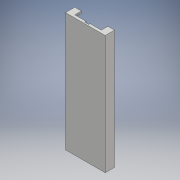
# Autodesk Inventor part: Base
Saved by Autodesk Inventor 2017 (Build 210142000, 142)
## iProperties
Created: 2017-01-18
Part Number: Base
Material: Generic
Document SubType Name: Modeling
Designer: A. Matías Quezada
Density: 1 g/cm^3
Appearance: Default
Author: A. Matías Quezada
Autodesk Inventor part; units mm, degrees
ref_plane "YZ Plane" through (0, 0, 0) normal (1, 0, 0) x (0, 1, 0)
ref_plane "XZ Plane" through (0, 0, 0) normal (0, 1, 0) x (-1, 0, 0)
ref_plane "XY Plane" through (0, 0, 0) normal (0, 0, 1) x (1, 0, 0)
sketch "Sketch1" plane through (0, 0, 0) normal (0, 1, 0) x (-1, 0, 0)
  line L0 (0, 0) -> (60, 0)
  line L1 (60, 0) -> (60, 180)
  line L2 (60, 180) -> (0, 180)
  line L3 (0, 180) -> (0, 0)
  dimension "d1" = 60
  dimension "d2" = 180
  constraints: 8 end point, 2 parallel, 1 horizontal, 1 perpendicular
  measures "d1" distance of L2.end L1.end
  measures "d2" distance of L1.end L0.end
extrude "Base" add sketch "Sketch1" along normal blind 4
sketch "Sketch3" plane through (0, 4, 0) normal (0, 1, 0) x (1, 0, 0)
  line L0 (-60, 0) -> (-60, -180) projected
  line L1 (-60, -180) -> (0, -180) projected
  line L2 (0, -180) -> (0, 0) projected
  line L3 (0, 0) -> (-60, 0) projected
  line L4 (-57, -177) -> (-57, -3)
  line L5 (-57, -3) -> (-3, -3)
  line L6 (-3, -3) -> (-3, -177)
  line L7 (-3, -177) -> (-57, -177)
  line L8 (-30, -198.6939) -> (-30, 11.8917)
  line L9 (-50, -180) -> (-10, -180)
  line L10 (-10, -180) -> (-10, -177)
  line L11 (-10, -177) -> (-50, -177)
  line L12 (-50, -177) -> (-50, -180)
  point P0 (-30, 0)
  point P1 (-30, -180)
  point P2 (-30, -177)
  dimension "d10" = 3
  dimension "d11" = 40
  constraints: 18 end point, 5 midpoint, 2 parallel, 1 horizontal, 1 perpendicular, 1 point on line, 1 vertical, 3 other
  measures "d10" distance between parallel lines of L0 L4
  measures "d11" distance between parallel lines of L10 L12
extrude "Muros" add sketch "Sketch3" along normal blind 10 contours L3 L8 L5 L4 L7 L12 L1 L0 | L3 L2 L1 L10 L7 L6 L5 L8
sketch "Sketch4" plane through (0, 4, 0) normal (0, 1, 0) x (1, 0, 0)
  line L0 (-50, -180) -> (-10, -180) projected
  line L1 (-57, -3) -> (-3, -3) projected
  line L2 (-33, -180) -> (-27, -180)
  line L3 (-27, -180) -> (-27, -3)
  line L4 (-27, -3) -> (-33, -3)
  line L5 (-33, -3) -> (-33, -180)
  line L6 (-3, -3) -> (-57, -3) projected
  point P0 (0, 0)
  point P1 (-30, -3)
  point P2 (-30, -3)
  point P3 (-30, -180)
  dimension "d14" = 6
  constraints: 8 end point, 5 midpoint, 2 parallel, 1 horizontal, 1 perpendicular
  measures "d14" distance between parallel lines of L3 L5
extrude "Rail" cut sketch "Sketch4" against normal blind 2
equation "\"d1\" = base_base_ancho"
equation "\"d2\" = base_base_largo"
equation "\"d4\" = base_base_grosor"
equation "\"d10\" = base_muros_grosor"
equation "\"d11\" = base_muros_separación"
equation "\"d12\" = base_muros_alto"
equation "\"d14\" = base_rail_ancho"
equation "\"d15\" = base_rail_profundidad"
equation "\"base_base_ancho\" = 60"
equation "\"base_base_largo\" = 180"
equation "\"base_base_grosor\" = 4"
equation "\"base_muros_grosor\" = 3"
equation "\"base_muros_separación\" = 40"
equation "\"base_muros_alto\" = 10"
equation "\"base_rail_ancho\" = 6"
equation "\"base_rail_profundidad\" = 2"
body "Solid1"
